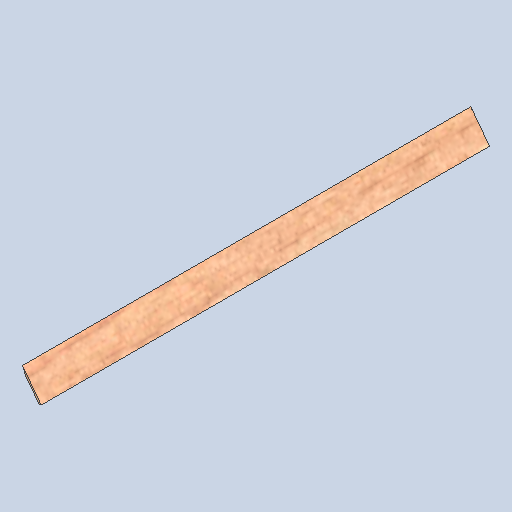
# Autodesk Inventor part: 2P.03.01.05.IM.FlapCutFill
Saved by Autodesk Inventor 2025.2 (Build 292293000, 293)
## iProperties
Created: 2025-01-05
Part Number: 2P.03.01.05.IM.FlapCutFill
Material: Wood (Birch)
Document SubType Name: Modeling
Designer: Imist
Density: 0.55 g/cm^3
Appearance: Birch - Natural Polished
Author: Imist
Autodesk Inventor part; units mm, degrees
ref_plane "YZ Plane" through (0, 0, 0) normal (1, 0, 0) x (0, 1, 0)
ref_plane "XZ Plane" through (0, 0, 0) normal (0, 1, 0) x (-1, 0, 0)
ref_plane "XY Plane" through (0, 0, 0) normal (0, 0, 1) x (1, 0, 0)
sketch "Sketch2" plane through (0, 0, 0) normal (0, 0, 1) x (1, 0, 0)
  line L0 (0.8995, 1.7758) -> (0.8995, 1.7675)
  line L1 (0.0945, 4.1741) -> (8.121, -6.4816)
  line L2 (0.8995, 1.7758) -> (7.1773, -6.5584)
  line L3 (7.1773, -6.5584) -> (8.121, -6.4816)
  arc A0 (0.8995, 1.7675) -> (0.0945, 4.1741) centre (-3.1005, 1.7675) ccw
  point P0 (0, 0)
  point P1 (1.9373, -6.9846)
  point P2 (6.534, -6.6107)
  dimension "d7" = 0.8
  constraints: 8 end point, 2 point on circle, 2 tangent, 1 centre point, 1 parallel, 1 point on line, 1 vertical
  measures "d7" distance between parallel lines of L1 L2
extrude "Extrusion2" add sketch "Sketch2" along normal blind 192
body "Solid2"
